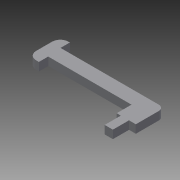
# Autodesk Inventor part: Gripper V 8.0 servo bracket side left 3mm
Saved by Autodesk Inventor 2015 (Build 190159000, 159)
## iProperties
Created: 2015-06-23
Part Number: Gripper V 8.0 servo bracket side left 3mm
Material: Generic
Document SubType Name: Modeling
Designer: Stackpole
Density: 1 g/cm^3
Appearance: Default
Author: Stackpole
Autodesk Inventor part; units mm, degrees
ref_plane "YZ Plane" through (0, 0, 0) normal (1, 0, 0) x (0, 1, 0)
ref_plane "XZ Plane" through (0, 0, 0) normal (0, 1, 0) x (-1, 0, 0)
ref_plane "XY Plane" through (0, 0, 0) normal (0, 0, 1) x (1, 0, 0)
sketch "Sketch1" plane through (0, 0, 0) normal (0, 0, 1) x (1, 0, 0)
  line L0 (0.039, 0.2446) -> (0.039, 3.6446)
  line L1 (-3.961, 12.0746) -> (-3.961, 0.2446)
  line L2 (-3.961, 0.2446) -> (0.039, 0.2446)
  line L3 (6.039, 3.6446) -> (30.489, 3.6446)
  line L4 (-3.961, 12.0746) -> (-0.45, 12.0746)
  line L5 (-0.45, 12.0746) -> (-0.45, 8.6446)
  line L6 (0.039, 3.6446) -> (6.039, 3.6446)
  line L7 (-0.45, 8.6446) -> (37.489, 8.6446)
  line L8 (30.489, 3.6446) -> (30.489, -1.7694)
  line L9 (37.489, -1.7694) -> (37.489, 8.6446)
  line L10 (30.489, -1.7694) -> (32, -1.7694)
  line L11 (32, -1.7694) -> (32, -7.6694)
  line L12 (32, -7.6694) -> (35, -7.6694)
  line L13 (35, -7.6694) -> (35, -1.7694)
  line L14 (35, -1.7694) -> (37.489, -1.7694)
  dimension "d0" = 6
  dimension "d10" = 4
  dimension "d22" = 3.4
  dimension "d23" = 3.43
  dimension "d24" = 5
  dimension "d25" = 24.45
  dimension "d26" = 7
  dimension "d31" = 5.9
  dimension "d32" = 3
  dimension "d33" = 1.511
  dimension "d36" = 5.414
  constraints: 30 end point, 8 perpendicular, 5 horizontal, 2 vertical, 1 point on line
  measures "d0" distance of L3.start L0.end
  measures "d10" distance of L1.end L0.start
  measures "d22" distance of L0.start L0.end
  measures "d23" distance of L4.end L5.end
  measures "d24" distance between parallel lines of L6 L7
  measures "d25" distance of L3.start L3.end
  measures "d26" distance of L8.end L9.start
  measures "d31" distance of L12.end L13.end
  measures "d32" distance of L11.end L12.end
  measures "d33" distance of L8.end L10.end
  measures "d36" distance between parallel lines of L10 L3
extrude "Extrusion1" add sketch "Sketch1" along normal blind 3
fillet "Fillet5" radius 2 1 edges at (37.489, 8.6446, 1.5)
fillet "Fillet6" radius 3 2 edges at (-3.961, 12.0746, 1.5) (-3.961, 0.2446, 1.5)
body "Solid1"
